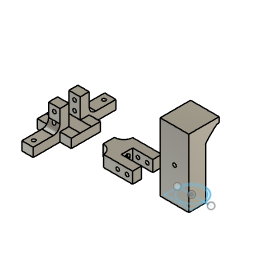
Load cell stand (Autodesk Fusion 360 design; units mm, degrees)
Autodesk Fusion 360 part; units mm, degrees
note: some values were not read from the file. Chosen so that the rebuilt part matches the saved one: which face or edge a step refers to; which pieces of a blend or face edit are solid.
sketch "Sketch1" plane through (0, 0, 0) normal (0, 0, 1) x (1, 0, 0)
  line L0 (0, 0) -> (12.67, 0)
  line L1 (12.67, 0) -> (12.67, 12.67)
  line L2 (12.67, 12.67) -> (0, 12.67)
  line L3 (0, 12.67) -> (0, 0)
  dimension "d1" = 12.67
  dimension "d2" = 12.67
  constraint horizontal L0
  constraint vertical L1
  constraint horizontal L2
  constraint vertical L3
  constraint coincident L0.start L3.end
  measures "d1" distance of L0.start L0.end
  measures "d2" distance of L0.start L2.end
extrude "Extrude1" add sketch "Sketch1" along normal blind 75.2 makes body 1
sketch "Sketch3" plane through (0, 0, 0) normal (-1, 0, 0) x (0, -1, 0)
  line L0 (-12.67, 0) -> (0, 0)
  line L1 (0, 0) -> (0, 75.2)
  line L2 (0, 75.2) -> (-12.67, 75.2)
  line L3 (-12.67, 75.2) -> (-12.67, 0)
  line L4 (-6.335, 0) -> (-6.335, 4.16) construction
  line L5 (-6.335, 4.16) -> (0, 4.16) construction
  line L6 (-6.335, 4.16) -> (-12.67, 4.16) construction
  line L7 (-12.67, 4.16) -> (-8.34, 4.16) construction
  line L8 (-8.34, 4.16) -> (-8.34, 8.17) construction
  line L9 (0, 4.16) -> (-4.33, 4.16) construction
  line L10 (-4.33, 4.16) -> (-4.33, 8.17) construction
  circle A0 centre (-6.335, 6.165) radius 2.005
  line L11 (-8.34, 8.17) -> (-4.33, 8.17)
  line L12 (-8.34, 8.17) -> (-8.34, 14.71) construction
  line L13 (-4.33, 8.17) -> (-4.33, 14.71) construction
  line L14 (-8.34, 14.71) -> (-4.33, 14.71) construction
  line L15 (-8.34, 14.71) -> (-8.34, 21.4984) construction
  line L16 (-4.33, 14.71) -> (-4.33, 21.3782) construction
  circle A1 centre (-6.335, 16.715) radius 2.005
  line L17 (-12.67, 37.6) -> (0, 37.6) construction
  circle A2 centre (-6.335, 58.485) radius 2.005
  circle A3 centre (-6.335, 69.035) radius 2.005
  line L18 (-6.335, 0) -> (-6.335, 18.72) construction
  line L19 (-6.335, 18.72) -> (0, 18.72) construction
  line L20 (0, 18.72) -> (0, 24.72) construction
  line L21 (0, 24.72) -> (-12.67, 24.72) construction
  dimension "d5" = 4.16
  dimension "d6" = 4.33
  dimension "d7" = 4.33
  dimension "d8" = 6.54
  dimension "d9" = 6.54
  dimension "d20" = 4.01
  dimension "d28" = 6
  constraint midpoint L0 L4.start
  constraint perpendicular L0 L4
  constraint coincident L1 L5.end
  constraint perpendicular L1 L5
  constraint coincident L3 L6.end
  constraint perpendicular L3 L6
  constraint perpendicular L3 L7
  constraint perpendicular L6 L8
  constraint perpendicular L1 L9
  constraint perpendicular L5 L10
  constraint tangent L8 A0
  constraint tangent L5 A0
  constraint tangent L10 A0
  constraint perpendicular L10 L11
  constraint tangent A0 L11
  constraint perpendicular L11 L12
  constraint perpendicular L11 L13
  constraint perpendicular L14 L15
  constraint perpendicular L14 L16
  constraint tangent L15 A1
  constraint tangent L14 A1
  constraint tangent L16 A1
  constraint midpoint L3 L17.start
  constraint midpoint L1 L17.end
  constraint symmetric A0 L17 A3
  constraint symmetric A1 L17 A2
  constraint coincident A1 L18.end
  constraint perpendicular L14 L18
  constraint coincident L1 L19.end
  constraint tangent A1 L19
  constraint perpendicular L19 L20
  constraint coincident L3 L21.end
  constraint perpendicular L3 L21
  measures "d5" distance of L4.start L4.end
  measures "d6" distance of L6.end L7.end
  measures "d7" distance of L5.end L9.end
  measures "d8" distance of L8.end L12.end
  measures "d9" distance of L10.end L13.end
  measures "d20" diameter of A3
  measures "d28" distance of L19.end L20.end
extrude "Extrude2" cut sketch "Sketch3" against normal blind 15 contours A0 | A1 | A2 | A3 bodies 1
sketch "Sketch4" plane through (0, 0, 0) normal (0, 0, 1) x (1, 0, 0)
  circle A0 centre (43, 13) radius 12.7
  line L0 (43, 13) -> (65, 13)
  line L1 (43, 13) -> (27, 13)
  line L2 (28, 13) -> (28, -2)
  line L3 (28, -2) -> (58, -2)
  line L4 (58, -2) -> (58, 13)
  arc A1 (58, 13) -> (28, 13) centre (43, 13) ccw
  dimension "d14" = 25.4
  dimension "d15" = 30
  constraint concentric A0 A1
  constraint coincident A0.centre L0.start
  constraint horizontal L0
  constraint parallel L0 L1
  constraint coincident L1 L2.start
  constraint perpendicular L1 L2
  constraint perpendicular L2 L3
  constraint coincident L0 L4.end
  constraint tangent L4 A1
  constraint tangent L3 A1
  measures "d14" diameter of A0
  measures "d15" diameter of A1
extrude "Extrude3" add sketch "Sketch4" along normal blind 70 separate body contours A0 L0 L1 L2 L3 L4 makes body 2
sketch "Sketch5" plane through (0, 0, 70) normal (0, 0, 1) x (-1, 0, 0)
  line L0 (-30.3, -13) -> (-28, -13)
  line L1 (-28, -13) -> (-28, 2)
  line L2 (-28, 2) -> (-58, 2)
  line L3 (-58, 2) -> (-58, -13)
  line L4 (-58, -13) -> (-55.7, -13)
  arc A0 (-30.3, -13) -> (-55.7, -13) centre (-43, -13) ccw
  line L5 (-28, -13) -> (-28, -28)
  line L6 (-28, -28) -> (-58, -28)
  line L7 (-58, -28) -> (-58, -13)
  constraint coincident L0.end L1.start
  constraint perpendicular L0 L5
  constraint perpendicular L5 L6
  constraint coincident L3.end L4.start
  constraint parallel L3 L7
extrude "Extrude4" add sketch "Sketch5" along normal blind 6 bodies 2
sketch "Sketch6" plane through (0, -2, 0) normal (0, -1, 0) x (1, 0, 0)
  line L0 (28, 0) -> (58, 0)
  line L1 (58, 0) -> (58, 76)
  line L2 (58, 76) -> (28, 76)
  line L3 (28, 76) -> (28, 0)
  line L4 (28, 38) -> (58, 38) construction
  circle A0 centre (43, 38) radius 2
  dimension "d21" = 4
  constraint midpoint L3 L4.start
  constraint midpoint L1 L4.end
  constraint midpoint L4 A0.centre
  measures "d21" diameter of A0
extrude "Extrude5" cut sketch "Sketch6" against normal blind 15 contours A0 bodies 2
ref_plane "WorkPlane1" through (43, 0.3, 38) normal (0, -1, 0) x (1, 0, 0)
sketch "Sketch7" plane through (0, 0.3, 0) normal (0, -1, 0) x (-1, 0, 0)
  circle A0 centre (-43, -38) radius 3
  dimension "d25" = 6
  measures "d25" diameter of A0
extrude "Extrude6" cut sketch "Sketch7" against normal blind 4 bodies 2
move_face "OffsetFaces1" offset 4 1 faces at (42.9502, -2, 63.9981) on bodies 2
extrude "Extrude12" cut 1 faces at (45.6611, 0.3, 38) along direction (0, -1, 0) blind 3.25 on bodies 2 bodies 2
sketch "Sketch8" plane through (0, 0, 0) normal (0, 0, 1) x (1, 0, 0)
  line L0 (0, 12.67) -> (-22.5, 12.67)
  line L1 (-22.5, 22.67) -> (0, 22.67)
  line L2 (0, 22.67) -> (0, 12.67)
  line L3 (0, 0) -> (-22.5, 0)
  line L4 (-22.5, -10) -> (0, -10)
  line L5 (0, -10) -> (0, 0)
  line L6 (-22.5, 22.67) -> (-32.5, 22.67)
  line L7 (-32.5, -10) -> (-22.5, -10)
  line L8 (-22.5, 0) -> (-22.5, 12.67)
  line L9 (0, 12.67) -> (-43, 12.67) construction
  line L10 (0, 0) -> (-43, 0) construction
  line L11 (-43, 12.67) -> (-43, 0)
  line L12 (-43, 12.67) -> (-32.5, 12.67)
  line L13 (-32.5, 0) -> (-43, 0)
  line L14 (-32.5, 22.67) -> (-32.5, 12.67)
  line L15 (-32.5, 0) -> (-32.5, -10)
  point P0 (0, 12.67)
  dimension "d29" = 22.5
  dimension "d30" = 10
  dimension "d31" = 22.5
  dimension "d32" = 10
  dimension "d33" = 10
  dimension "d34" = 43
  constraint horizontal L0
  constraint horizontal L1
  constraint vertical L2
  constraint coincident P0 L0.start
  constraint horizontal L3
  constraint horizontal L4
  constraint vertical L5
  constraint coincident L3.start L5.end
  constraint horizontal L6
  constraint vertical L14
  constraint horizontal L7
  constraint vertical L8
  constraint perpendicular L9 L14
  constraint perpendicular L5 L10
  constraint coincident L9 L12.end
  constraint coincident L13.start L14
  constraint coincident L10 L13.start
  constraint collinear L14 L15
  measures "d29" distance of P0 L0.end
  measures "d30" distance of P0 L1.end
  measures "d31" distance of L3.start L3.end
  measures "d32" distance of L3.start L4.end
  measures "d33" distance of L1.start L6.end
  measures "d34" distance of P0 L9.end
extrude "Extrude7" add sketch "Sketch8" along normal blind 12.67 separate body makes body 3
sketch "Sketch9" plane through (0, -10, 0) normal (0, -1, 0) x (1, 0, 0)
  line L0 (-32.5, 0) -> (0, 0)
  line L1 (0, 0) -> (0, 12.67)
  line L2 (0, 12.67) -> (-32.5, 12.67)
  line L3 (-32.5, 12.67) -> (-32.5, 0)
  line L4 (-22.5, 12.67, -10) -> (-22.5, 12.67, 0) construction
  line L5 (-22.5, 12.67) -> (-22.5, 0) construction
  line L6 (-14.7124, 8.2632) -> (-8.1724, 8.2632) construction
  line L7 (-14.7124, 8.2632) -> (-14.7124, 4.3657)
  line L8 (-18.61, 12.5932) -> (-18.6043, 8.2632) construction
  line L9 (-22.5037, 12.6493) -> (-22.4963, -0.0207)
  line L10 (-18.6064, 4.3657) -> (-14.7124, 4.3657) construction
  line L11 (-18.61, 0.0357) -> (-18.6064, 4.3657) construction
  line L12 (-18.61, 6.3166) -> (-18.61, 12.5932) construction
  line L13 (-18.6043, 8.2632) -> (-14.7124, 8.2632) construction
  circle A0 centre (-6.1674, 6.3143) radius 2.005
  line L14 (-18.61, 6.3166) -> (-18.61, 0.0357) construction
  line L15 (-22.5, 6.3143) -> (-18.61, 6.3166) construction
  line L16 (-8.1724, 8.2632) -> (-8.1724, 4.3657) construction
  line L17 (-22.5, 6.3143) -> (-4.1624, 6.3143) construction
  line L18 (-14.7124, 4.3657) -> (-8.1724, 4.3657) construction
  circle A1 centre (-16.6612, 6.3145) radius 1.9488
  point P0 (-22.5, 12.67)
  point P1 (-22.5, 0)
  dimension "d37" = 3.89
  dimension "d38" = 4.33
  dimension "d39" = 4.33
  dimension "d40" = 6.54
  dimension "d41" = 6.54
  dimension "d55" = 4.01
  constraint coincident P0 L5.start
  constraint coincident L2 P0
  constraint coincident L0 P1
  constraint perpendicular L0 L5
  constraint midpoint L15.start L9
  constraint perpendicular L9 L15
  constraint perpendicular L12 L13
  constraint perpendicular L10 L14
  constraint tangent L13 A1
  constraint tangent L14 A1
  constraint tangent L10 A1
  constraint perpendicular L7 L10
  constraint perpendicular L6 L7
  constraint perpendicular L7 L18
  constraint tangent A0 L16
  constraint coincident L17.end A0
  constraint perpendicular L16 L17
  constraint perpendicular L2 L12
  constraint tangent L7 A1
  constraint coincident A0.centre L17
  measures "d37" distance of L15.start L12.start
  measures "d38" distance of L8.start L8.end
  measures "d39" distance of L11.start L10.start
  measures "d40" distance of L6.start L6.end
  measures "d41" distance of L7.end L16.end
  measures "d55" diameter of A0
extrude "Extrude8" cut sketch "Sketch9" against normal blind 38 contours A0 | A1 bodies 3
sketch "Sketch10" plane through (-43, 0, 0) normal (-1, 0, 0) x (0, -1, 0)
  line L0 (-12.67, 0) -> (0, 0)
  line L1 (0, 0) -> (0, 12.67)
  line L2 (0, 12.67) -> (-12.67, 12.67)
  line L3 (-12.67, 12.67) -> (-12.67, 0)
  line L4 (-6.335, 0) -> (-6.335, 12.67) construction
  line L5 (0, 6.335) -> (-12.67, 6.335) construction
  circle A0 centre (-6.335, 6.335) radius 2
  dimension "d44" = 4
  constraint midpoint L0 L4.start
  constraint midpoint L2 L4.end
  constraint midpoint L1 L5.start
  constraint midpoint L3 L5.end
  constraint midpoint L5 A0.centre
  measures "d44" diameter of A0
copy_body "CopyPasteBodies2" bodies 3 makes body 4
move_body "Move2" bodies 4 to x (1, 0, 0) y (0, 1, 0) z (0, 0, 1) at (-60, 0, 0)
extrude "Extrude9" cut sketch "Sketch10" against normal blind 15 contours A0 bodies 3
extrude "Extrude10" cut 1 faces at (-99.5, 12.67, 4.2233) along direction (0, -1, 0) blind 18 on bodies 4 bodies 4
move_body "Move3" bodies 4 to x (0, 0, 1) y (0, 1, 0) z (-1, 0, 0) at (-81.3377, 0, 95.7759)
move_body "Move4" bodies 4 to x (1, 0, 0) y (0, 1, 0) z (0, 0, 1) at (0, 0, -3)
sketch "Sketch12" plane through (-94.0077, 0, 0) normal (-1, 0, 0) x (0, -1, 0)
  line L0 (-22.67, 0.2759) -> (10, 0.2759)
  line L1 (10, 0.2759) -> (10, 32.7759)
  line L2 (10, 32.7759) -> (0, 32.7759)
  line L3 (0, 32.7759) -> (0, 10.2759)
  line L4 (0, 10.2759) -> (-12.67, 10.2759)
  line L5 (-12.67, 10.2759) -> (-12.67, 32.7759)
  line L6 (-12.67, 32.7759) -> (-22.67, 32.7759)
  line L7 (-22.67, 32.7759) -> (-22.67, 0.2759)
  line L8 (0, 10.2759) -> (10, 10.2759)
  line L9 (-12.67, 10.2759) -> (-22.67, 10.272)
  constraint coincident L3.end L4.start
  constraint coincident L1 L8.end
  constraint perpendicular L1 L8
  constraint coincident L4.end L5.start
  constraint coincident L7 L9.end
extrude "Extrude13" add sketch "Sketch12" along normal blind 12.67 contours L0 L1 L4 L7 L8 L9 bodies 4
extrude "Extrude14" add 1 faces at (-106.6777, 4.2233, 3.6093) along direction (1, 0, 0) blind 38.01 on bodies 4 bodies 4
sketch "Sketch13" plane through (0, -10, 0) normal (0, -1, 0) x (1, 0, 0)
  line L0 (-81.3377, 10.2759) -> (-81.3377, 32.7759)
  line L1 (-81.3377, 32.7759) -> (-94.0077, 32.7759)
  line L2 (-94.0077, 32.7759) -> (-94.0077, 10.2759)
  line L3 (-94.0077, 10.2759) -> (-94.0077, 0.2759)
  line L4 (-94.0077, 0.2759) -> (-81.3377, 0.2759)
  line L5 (-81.3377, 0.2759) -> (-81.3377, 10.2759)
  circle A0 centre (-87.6522, 16.1147) radius 1.9488
  circle A1 centre (-87.652, 26.6085) radius 2.005
  line L6 (-106.6777, 10.2759) -> (-68.6677, 10.2759)
  point P0 (-106.6777, 10.2759)
  point P1 (-68.6677, 10.2759)
  constraint coincident P0 L6.start
  constraint coincident P1 L6.end
extrude "Extrude15" add sketch "Sketch13" along normal blind 30 contours L3 L4 L5 L6 bodies 4
extrude "Extrude16" add 1 faces at (-89.7844, -40, 6.9426) along direction (0, 1, 0) blind 92.67 on bodies 4 bodies 4
fillet "Fillet1" radius 7.5 1 edges at (-87.6727, 22.67, 10.2759) on bodies 4
fillet "Fillet2" radius 7.5 1 edges at (-87.6727, -10, 10.2759) on bodies 4
fillet "Fillet3" radius 10.5 2 edges at (-32.5, 0, 6.335) (-32.5, 12.67, 6.335) on bodies 3
move_face "OffsetFaces2" offset 1 1 faces at (58, 0.3333, 48.6667) on bodies 2
move_face "OffsetFaces3" offset 1 2 faces at (28, 0.3333, 48.6667) (28, 18, 72) on bodies 2
fillet "Fillet4" radius 12.7 tangency weight 0.1 2 edges at (28.65, 13, 70) (57.35, 13, 70) on bodies 2
extrude "Extrude17" cut 1 faces at (-28, 6.6683, 6.9124) along direction (1, 0, 0) blind 15 on bodies 3 bodies 3
sketch "Sketch14" plane through (-22.5, 0, 0) normal (1, 0, 0) x (0, 1, 0)
  circle A0 centre (6.335, 6.335) radius 2
  line L0 (0, 0) -> (12.67, 0)
  line L1 (12.67, 0) -> (12.67, 12.67)
  line L2 (12.67, 12.67) -> (0, 12.67)
  line L3 (0, 12.67) -> (0, 0)
  line L4 (6.335, 10.085) -> (3.0874, 8.21)
  line L5 (3.0874, 8.21) -> (3.0874, 4.46)
  line L6 (3.0874, 4.46) -> (6.335, 2.585)
  line L7 (6.335, 2.585) -> (9.5826, 4.46)
  line L8 (9.5826, 4.46) -> (9.5826, 8.21)
  line L9 (9.5826, 8.21) -> (6.335, 10.085)
  point P0 (6.335, 6.335)
  dimension "d76" = 3.75
  constraint coincident P0 A0.centre
  measures "d76" distance of L4.start P0
extrude "Extrude18" cut sketch "Sketch14" against normal blind 3 contours L4 L5 L6 L7 L8 L9 bodies 3
ref_plane "WorkPlane2" through (-87.6727, 22.67, 21.5259) normal (0, -1, 0) x (0, 0, 1)
sketch "Sketch15" plane through (0, 0, 10.2759) normal (0, 0, 1) x (-1, 0, 0)
  line L0 (94.0077, -30.17) -> (81.3377, -30.17)
  line L1 (81.3377, -30.17) -> (81.3377, -52.67)
  line L2 (81.3377, -52.67) -> (94.0077, -52.67)
  line L3 (94.0077, -52.67) -> (94.0077, -30.17)
  circle A0 centre (87.6727, -45.67) radius 2
  circle A1 centre (87.6727, 33) radius 2
  line L4 (81.3377, 40) -> (94.0077, 40) construction
  point P0 (87.6727, -52.67)
  point P1 (87.6727, 40)
  dimension "d80" = 4
  dimension "d81" = 7
  dimension "d82" = 4
  dimension "d83" = 7
  constraint midpoint L2 P0
  constraint vertical A0.centre P0
  constraint midpoint L4 P1
  constraint vertical A1.centre P1
  measures "d80" diameter of A0
  measures "d81" distance of L2 A0.centre
  measures "d82" diameter of A1
  measures "d83" distance of A1.centre L4
extrude "Extrude19" cut sketch "Sketch15" against normal blind 21 contours A0 | A1 bodies 4
hidden bodies 1
equation "d6 = 4.83 mm - 0.5 mm"
equation "d7 = 4.83 mm - 0.5 mm"
equation "d34 = 33 mm + 10 mm"
equation "d38 = 4.83 mm - 0.5 mm"
equation "d39 = 4.83 mm - 0.5 mm"
equation "d58 = -12.67 * 3 mm"
equation "d62 = -32.67 mm - 30 mm - 30 mm"
equation "d76 = ( 7.5 / 2 ) * 1 mm"
